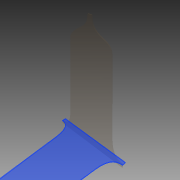
# Autodesk Inventor part: Plate
Saved by Autodesk Inventor 2012 (Build 160160000, 160)
## iProperties
Created: 2013-02-28
Part Number: Plate
Material: High Impact Polystyrene
Document SubType Name: Modeling
Designer: fixer
Mass: 195.332 g
Surface Area: 1241.74 cm^2
Volume: 191.127 cm^3
Density: 1.022 g/cm^3
Author: fixer
Autodesk Inventor part; units mm, degrees
ref_plane "YZ Plane" through (0, 0, 0) normal (1, 0, 0) x (0, 1, 0)
ref_plane "XZ Plane" through (0, 0, 0) normal (0, 1, 0) x (-1, 0, 0)
ref_plane "XY Plane" through (0, 0, 0) normal (0, 0, 1) x (1, 0, 0)
sketch "Sketch1" plane through (0, 0, 0) normal (0, 0, 1) x (1, 0, 0)
  line L0 (76.2, -12.7) -> (381, -12.7) construction
  line L1 (-76.2, -12.7) -> (-381, -12.7) construction
  line L2 (-76.2, 0) -> (-381, 0) construction
  line L3 (76.2, 0) -> (381, 0) construction
  line L4 (0, -116.2267) -> (0, 608.4603)
  line L5 (0, -12.7) -> (-130.6862, -12.7)
  line L6 (-130.6862, -12.7) -> (-130.6862, 0)
  line L7 (0, 394.3626) -> (-6.35, 394.3626)
  line L8 (-68.9484, 319.31) -> (-84.1436, 93.9477)
  spline S0 degree 3 poles (-130.6862, 0) (-85.9047, 0) (-86.5842, 57.7519) (-84.1436, 93.9477) knots 0 0 0 0 1 1 1 1
  line L9 (-134.8846, 0) -> (-126.4878, 0) construction
  arc A0 (-134.0379, 0.108) -> (-127.3344, 0.108) centre (-130.6862, 52.086) ccw construction
  line L10 (68.9484, 319.31) -> (84.1436, 93.9477)
  line L11 (0, 394.3626) -> (6.35, 394.3626)
  spline S1 degree 3 poles (130.6862, 0) (85.9047, 0) (86.5842, 57.7519) (84.1436, 93.9477) knots 0 0 0 0 1 1 1 1
  line L12 (134.8846, 0) -> (126.4878, 0) construction
  arc A1 (127.3344, 0.108) -> (134.0379, 0.108) centre (130.6862, 52.086) ccw construction
  line L13 (0, -12.7) -> (130.6862, -12.7)
  line L14 (130.6862, -12.7) -> (130.6862, 0)
  spline S2 degree 4 poles (-6.35, 394.3626) (-6.35, 368.2666) (-34.2436, 358.4082) (-52.0649, 343.9213) (-68.2317, 329.9384) (-68.9484, 319.31) knots 0 0 0 0 0 0.532569 1 1 1 1 1
  line L15 (-6.35, 421.2444) -> (-6.35, 367.4808) construction
  arc A2 (-9.8147, 374.0762) -> (-9.8147, 414.649) centre (-67.4729, 394.3626) ccw construction
  spline S3 degree 4 poles (6.35, 394.3626) (6.35, 345.3624) (45.5969, 356.9185) (67.4153, 342.0479) (68.9484, 319.31) knots 0 0 0 0 0 1 1 1 1 1
  line L16 (6.35, 421.2444) -> (6.35, 367.4808) construction
  arc A3 (9.8147, 414.649) -> (9.8147, 374.0762) centre (67.4729, 394.3626) ccw construction
  line L17 (-33.3575, 356.6691) -> (-58.9017, 338.5396) construction
  arc A4 (-35.6685, 354.4519) -> (-56.0459, 339.9893) centre (50.0086, 212.1476) ccw construction
  point P0 (0, 0)
  point P1 (-46.1296, 347.6043)
  point P2 (46.1296, 347.6043)
  dimension "d0" = 6.35
  constraints: 36 end point, 16 symmetric about line, 9 horizontal, 8 midpoint, 5 centre point, 5 point on circle, 5 point on line, 4 vertical, 2 perpendicular, 21 other
  measures "d0" distance of L7.start L7.end
extrude "Extrusion1" add sketch "Sketch1" against normal blind 3.175
body "Solid1"
